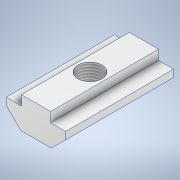
# Autodesk Inventor part: Pasador
Saved by Autodesk Inventor 2020.3 (Build 243373000, 373)
## iProperties
Created: 2020-12-09
Part Number: Pasador
Material: Aluminio 6061
Document SubType Name: Modeling
Designer: Cerberus 1S
Density: 2.7 g/cm^3
Appearance: Aluminio - Plano
Author: Cerberus 1S
Autodesk Inventor part; units mm, degrees
ref_plane "YZ Plane" through (0, 0, 0) normal (1, 0, 0) x (0, 1, 0)
ref_plane "XZ Plane" through (0, 0, 0) normal (0, 1, 0) x (-1, 0, 0)
ref_plane "XY Plane" through (0, 0, 0) normal (0, 0, 1) x (1, 0, 0)
sketch "Boceto1" plane through (0, 0, 0) normal (0, 0, 1) x (1, 0, 0)
  line L0 (0, 0) -> (-2.65, 2.65)
  line L1 (8.35, 2.65) -> (5.7, 0)
  line L2 (8.35, 4) -> (8.35, 2.65)
  line L3 (-2.65, 4) -> (8.35, 4)
  line L4 (-2.65, 2.65) -> (-2.65, 4)
  line L5 (5.7, 0) -> (0, 0)
  dimension "d1" = 11
  dimension "d2" = 5.7
  dimension "d5" = 2.65
  dimension "d6" = 2.65
  dimension "d7" = 4
  dimension "d9" = 45
  dimension "d10" = 45
  constraints: 12 end point, 1 horizontal, 1 parallel
  measures "d1" distance between parallel lines of L2 L4
  measures "d2" distance of L0.start L1.end
  measures "d5" distance from line of L0.start L4
  measures "d6" distance from line of L2 L1.end
  measures "d7" distance from line of L1.end L3
  measures "d9" angle of L5 L0
  measures "d10" angle of L5 L1
extrude "Extrusión1" add sketch "Boceto1" along normal blind 20
sketch "Boceto3" plane through (-2.65, 4, 0) normal (0, 1, 0) x (1, 0, 0)
  line L0 (11, 0) -> (0, 0) projected
  line L1 (8.2, 0) -> (2.8, 0)
  line L2 (2.8, 0) -> (2.8, -20)
  line L3 (2.8, -20) -> (8.2, -20)
  line L4 (8.2, -20) -> (8.2, 0)
  line L5 (11, -20) -> (0, -20) projected
  line L6 (11, 0) -> (11, -20) projected
  line L7 (0, 0) -> (0, -20) projected
  point P0 (2.65, 0)
  point P1 (5.5, -20)
  point P2 (2.8, 0)
  dimension "d20" = 2.8
  dimension "d21" = 2.8
  constraints: 8 end point, 2 midpoint, 2 parallel, 1 horizontal, 1 perpendicular, 1 point on line
  measures "d20" distance between parallel lines of L6 L4
  measures "d21" distance between parallel lines of L7 L2
extrude "Extrusión2" add sketch "Boceto3" along normal blind 1.8 contours L4 L3 L2 L0
sketch "Boceto4" plane through (-2.65, 5.8, 0) normal (0, 1, 0) x (1, 0, 0)
  line L0 (8.2, 0) -> (2.8, 0) projected
  line L1 (5.5, 0) -> (5.5, -20)
  line L2 (2.8, -20) -> (8.2, -20) projected
  line L3 (2.8, 0) -> (2.8, -20) projected
  line L4 (2.8, -10) -> (5.5, -10)
  point P0 (2.65, 0)
  constraints: 4 end point, 4 midpoint
hole "Agujero2" at (2.85, 5.8, 10) direction (0, -1, 0) diameter 4.4587 depth 10 thread size "M5x0.5" class "6H" standard "ANSI Metric M Profile"
